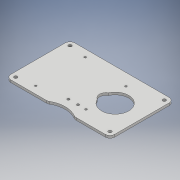
# Autodesk Inventor part: 06-01-Платформа для лидара
Saved by Autodesk Inventor 2018 (Build 220112000, 112)
## iProperties
Created: 2018-12-15
Part Number: 06-01-Платформа для лидара
Material: Типовые
Document SubType Name: Modeling
Designer: RR
Density: 1 g/cm^3
Appearance: По умолчанию
Author: RR
Autodesk Inventor part; units mm, degrees
ref_plane "YZ Plane" through (0, 0, 0) normal (1, 0, 0) x (0, 1, 0)
ref_plane "XZ Plane" through (0, 0, 0) normal (0, 1, 0) x (-1, 0, 0)
ref_plane "XY Plane" through (0, 0, 0) normal (0, 0, 1) x (1, 0, 0)
sketch "Эскиз1" plane through (0, 0, 0) normal (0, 0, 1) x (1, 0, 0)
  line L0 (-63, 0) -> (70, 0)
  line L1 (0, 29) -> (0, -30)
  circle A0 centre (35, 25) radius 1.25
  circle A1 centre (-22, 31) radius 1.25
  circle A2 centre (-22, -31) radius 1.25
  circle A3 centre (35, -25) radius 1.25
  arc A4 (31.0081, -7) -> (31.0081, 7) centre (46.5, 0) ccw
  line L2 (35, -25) -> (0, -25)
  circle A5 centre (25, -25) radius 1.5
  circle A6 centre (13, -25) radius 1.5
  arc A7 (31.0081, 7) -> (31.0081, -7) centre (35, 0) ccw
  line L3 (-44, 40) -> (74, 40)
  line L4 (80, 34) -> (80, -34)
  line L5 (-50, -34) -> (-50, 34)
  arc A8 (-44, 40) -> (-50, 34) centre (-44, 34) ccw
  arc A9 (-50, -34) -> (-44, -40) centre (-44, -34) ccw
  arc A10 (74, -40) -> (80, -34) centre (74, -34) ccw
  arc A11 (80, 34) -> (74, 40) centre (74, 34) ccw
  circle A12 centre (-44, 34) radius 2
  circle A13 centre (-44, -34) radius 2
  circle A14 centre (74, -34) radius 2
  circle A15 centre (74, 34) radius 2
  arc A16 (34.5621, -39.1892) -> (3.4379, -39.1892) centre (19, -66) ccw
  line L6 (74, -40) -> (37.5742, -40)
  line L7 (0.4258, -40) -> (-44, -40)
  arc A17 (0.4258, -40) -> (3.4379, -39.1892) centre (0.4258, -34) ccw
  arc A18 (34.5621, -39.1892) -> (37.5742, -40) centre (37.5742, -34) ccw
  point P0 (0, 0)
  point P1 (-50, 40)
  point P2 (80, 40)
  point P3 (80, -40)
  point P4 (-50, -40)
  point P5 (2.1181, -40)
  point P6 (35.8819, -40)
  dimension "d3" = 2.5
  dimension "d4" = 2.5
  dimension "d5" = 2.5
  dimension "d6" = 2.5
  dimension "d9" = 62
  dimension "d10" = 50
  dimension "d11" = 34
  dimension "d12" = 3
  dimension "d14" = 10
  dimension "d16" = 3
  dimension "d17" = 12
  dimension "d19" = 46.5
  dimension "d20" = 130
  dimension "d21" = 80
  dimension "d22" = 130
  dimension "d23" = 6
  dimension "d24" = 4
  dimension "d25" = 4
  dimension "d26" = 4
  dimension "d27" = 4
  dimension "d31" = 6
  constraints: 20 point on circle, 19 centre point, 16 end point, 14 tangent, 12 point on line, 4 coincident, 4 equal radius, 4 perpendicular, 2 horizontal, 1 vertical
  measures "d3" diameter of A0
  measures "d4" diameter of A1
  measures "d5" diameter of A2
  measures "d6" diameter of A3
  measures "d9" distance of A2.centre A1.centre
  measures "d10" distance of L2.start A0.centre
  measures "d11" diameter of A4
  measures "d12" diameter of A5
  measures "d14" distance of A5.centre L2.start
  measures "d16" diameter of A6
  measures "d17" distance of A5.centre A6.centre
  measures "d19" distance of A4.centre point (0, 0)
  measures "d20" distance of point (-50, 40) point (80, 40)
  measures "d21" distance of point (80, 40) point (80, -40)
  measures "d22" distance of point (80, -40) point (-50, -40)
  measures "d23" radius of A8
  measures "d24" diameter of A12
  measures "d25" diameter of A13
  measures "d26" diameter of A14
  measures "d27" diameter of A15
  measures "d31" radius of A17
extrude "Выдавливание1" add sketch "Эскиз1" along normal blind 3
